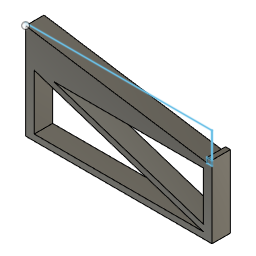
keybord_stand_v2 v1 (Autodesk Fusion 360 design; units mm, degrees)
Autodesk Fusion 360 part; units mm, degrees
sketch "Sketch6" plane through (0, 0, 0) normal (0, 1, 0) x (1, 0, 0)
  line L0 (0, 0) -> (152, 0)
  line L1 (152, 0) -> (152, -80)
  line L2 (152, -80) -> (0, -80)
  line L3 (0, -80) -> (0, 0)
  dimension "d14" = 152
  dimension "d15" = 80
  constraint horizontal L0
  constraint vertical L1
  constraint horizontal L2
  constraint vertical L3
  constraint coincident L0.start L3.end
  measures "d14" distance of L0.start L0.end
  measures "d15" distance of L0.start L2.end
extrude "Extrude5" add sketch "Sketch6" along normal blind 15 makes body 1
sketch "Sketch8" plane through (0, 0, 0) normal (0, 1, 0) x (1, 0, 0)
  line L0 (148, -55) -> (152, -55)
  line L1 (152, -55) -> (152, -59)
  line L2 (152, -59) -> (148, -59)
  line L3 (148, -59) -> (148, -55)
  line L4 (0, -78) -> (0, -80)
  line L5 (0, -80) -> (152, -80)
  line L6 (152, -80) -> (152, -59)
  line L7 (152, -59) -> (152, -80)
  dimension "d18" = 4
  dimension "d19" = 4
  constraint horizontal L0
  constraint vertical L1
  constraint horizontal L2
  constraint vertical L3
  constraint vertical L4
  constraint perpendicular L4 L5
  constraint perpendicular L5 L6
  measures "d18" distance of L0.start L0.end
  measures "d19" distance of L0.start L2.end
sketch "Sketch9" plane through (0, 0, 0) normal (0, -1, 0) x (1, 0, 0)
  line L0 (152, 80) -> (0, 80)
  line L1 (0, 80) -> (0, 0)
  line L2 (0, 0) -> (152, 0)
  line L3 (152, 0) -> (152, 80)
  line L4 (0, 54) -> (135, 54)
  line L5 (148, 55) -> (0, 78)
  line L6 (0, 80) -> (152, 80)
  line L7 (152, 59) -> (148, 59)
  line L8 (148, 59) -> (148, 55)
  line L9 (152, 59) -> (152, 80)
  constraint coincident L1 L4.start
  constraint coincident L1 L5.end
  constraint coincident L0.end L1.start
  constraint coincident L0.start L3.end
  constraint coincident L3 L7.start
  constraint perpendicular L3 L7
  constraint parallel L3 L8
extrude "Extrude7" cut sketch "Sketch9" against normal blind 15 contours L0 L1 L3 L5 L6 L7 L8 L9 bodies 1
sketch "Sketch10" plane through (0, 0, 0) normal (0, -1, 0) x (1, 0, 0)
  line L0 (152, 59) -> (148, 59)
  line L1 (148, 59) -> (148, 55)
  line L2 (148, 55) -> (0, 78)
  line L3 (0, 78) -> (0, 0)
  line L4 (0, 0) -> (152, 0)
  line L5 (152, 0) -> (152, 59)
  line L6 (145, 50) -> (7, 50)
  line L7 (7, 50) -> (7, 5)
  line L8 (7, 5) -> (145, 5)
  line L9 (145, 5) -> (145, 50)
  constraint horizontal L6
  constraint vertical L7
  constraint horizontal L8
  constraint vertical L9
extrude "Extrude8" cut sketch "Sketch10" against normal blind 15 contours L6 L7 L8 L9 bodies 1
sketch "Sketch11" plane through (0, 0, 0) normal (0, -1, 0) x (1, 0, 0)
  line L0 (7, 50) -> (145, 50)
  line L1 (145, 50) -> (145, 5)
  line L2 (145, 5) -> (7, 5)
  line L3 (7, 5) -> (7, 50)
  line L4 (152, 59) -> (148, 59)
  line L5 (148, 59) -> (148, 55)
  line L6 (148, 55) -> (0, 78)
  line L7 (0, 78) -> (0, 0)
  line L8 (0, 0) -> (152, 0)
  line L9 (152, 0) -> (152, 59)
  line L10 (7, 50) -> (145, 5)
  constraint coincident L0.start L3.end
  constraint coincident L1.end L2.start
surface "Extrude9" add extruded along (0, -1, 0) between 0 and -15 path "Sketch11" along L10 separate body makes body 2
extrude "Extrude10" add 1 faces at (99, 5, 20) along direction (0.310021, 0, 0.95073) blind 5 on bodies 2 bodies 1
extrude "Extrude6" [suppressed]
